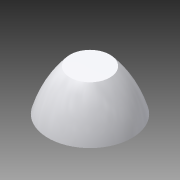
# Autodesk Inventor part: Head
Saved by Autodesk Inventor 2014 SP2 (Build 180246200, 246)
## iProperties
Created: 2014-09-17
Part Number: Head
Material: Polypropylene
Document SubType Name: Modeling
Designer: Sophiagirraffe
Density: 0.899 g/cm^3
Appearance: White
Author: Sophiagirraffe
Autodesk Inventor part; units mm, degrees
ref_plane "YZ Plane" through (0, 0, 0) normal (1, 0, 0) x (0, 1, 0)
ref_plane "XZ Plane" through (0, 0, 0) normal (0, 1, 0) x (-1, 0, 0)
ref_plane "XY Plane" through (0, 0, 0) normal (0, 0, 1) x (1, 0, 0)
sketch "Sketch1" plane through (0, 0, 0) normal (0, 0, 1) x (1, 0, 0)
  line L0 (0, 0) -> (0, 158.75)
  line L1 (0, 158.75) -> (76.2, 158.75)
  line L2 (0, 0) -> (160.3375, 0)
  arc A0 (160.3375, 0) -> (76.2, 158.75) centre (-236.7497, -108.7848) ccw
  dimension "d0" = 158.75
  dimension "d1" = 76.2
  dimension "d2" = 160.3375
  constraints: 6 end point, 2 point on circle, 1 centre point, 1 parallel, 1 perpendicular, 1 vertical
  measures "d0" distance of L0.start L0.end
  measures "d1" distance of L0.end L1.end
  measures "d2" distance of L0.start L2.end
revolve "Revolution1" add sketch "Sketch1" angle 360 about axis through (0, 0, 0) along (0, 1, 0)
shell "Shell1" thickness 5.08 removed faces 1 at (30.762, 0, 60.7873)
body "Solid1"
